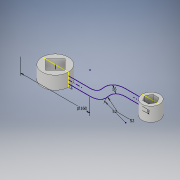
# Autodesk Inventor part: 練習三
Saved by Autodesk Inventor 2017 (Build 210142000, 142)
## iProperties
Part Number: 練習三
Material: 一般
Document SubType Name: Modeling
Designer: user
Density: 1 g/cm^3
Appearance: 預設
Author: user
Autodesk Inventor part; units mm, degrees
ref_plane "YZ Plane" through (0, 0, 0) normal (1, 0, 0) x (0, 1, 0)
ref_plane "XY Plane" through (0, 0, 0) normal (0, 0, 1) x (1, 0, 0)
sketch "草圖1" plane through (0, 0, 0) normal (0, 1, 0) x (-1, 0, 0)
  circle A0 centre (0, 0) radius 30
  line L0 (0, 22.6274) -> (-22.6274, 0)
  line L1 (-22.6274, 0) -> (0, -22.6274)
  line L2 (0, -22.6274) -> (22.6274, 0)
  line L3 (22.6274, 0) -> (0, 22.6274)
  line L4 (17.214, 3.8392) -> (-17.214, -3.8392) construction
  line L5 (-19.542, 13.3062) -> (19.542, -13.3062) construction
  line L6 (11.3137, -11.3137) -> (-26.3636, 26.3636)
  line L7 (-11.3137, -11.3137) -> (19.159, 19.159)
  dimension "d0" = 60
  dimension "d1" = 32
  dimension "d2" = 32
  constraints: 16 end point, 6 midpoint, 3 parallel, 3 point on line, 2 perpendicular, 1 centre point, 1 coincident, 1 other
  measures "d0" diameter of A0
  measures "d1" distance between parallel lines of L2 L0
  measures "d2" distance between parallel lines of L1 L3
extrude "擠出1" add sketch "草圖1" along normal blind 30
ref_plane "工作平面1" through (0, 71, 0) normal (0, 1, 0) x (1, 0, 0)
sketch "草圖2" plane through (0, 71, 0) normal (0, 1, 0) x (1, 0, 0)
  circle A0 centre (220, 0) radius 20
  line L0 (233.8564, 0) -> (226.9282, -12)
  line L1 (226.9282, -12) -> (213.0718, -12)
  line L2 (213.0718, -12) -> (206.1436, 0)
  line L3 (206.1436, 0) -> (213.0718, 12)
  line L4 (213.0718, 12) -> (226.9282, 12)
  line L5 (226.9282, 12) -> (233.8564, 0)
  point P0 (0, 0)
  dimension "d14" = 220
  dimension "d15" = 40
  dimension "d16" = 0
  dimension "d17" = 24
  constraints: 12 end point, 1 centre point, 1 coincident, 1 horizontal, 13 other
  measures "d14" distance of A0.centre point (0, 0)
  measures "d15" diameter of A0
  measures "d16" vertical distance of A0.centre point (0, 0)
  measures "d17" distance between parallel lines of L4 L1
extrude "擠出2" add sketch "草圖2" against normal blind 32
sketch "草圖3" plane through (0, 0, 0) normal (0, 0, 1) x (1, 0, 0)
  line L0 (-30, 0) -> (30, 0) projected
  line L1 (30, 7) -> (80, 7)
  line L2 (161.9756, 47) -> (200, 47)
  line L3 (200, 71) -> (200, 39) projected
  line L4 (200, 39) -> (240, 39) projected
  line L5 (30, 30) -> (-30, 30) projected
  line L6 (30, 0) -> (30, 30) projected
  line L7 (200, 71) -> (240, 71) projected
  arc A0 (161.9756, 47) -> (120.9878, 27) centre (161.9756, -5) ccw
  arc A1 (80, 7) -> (120.9878, 27) centre (80, 59) ccw
  line L8 (30, 15) -> (64.6593, 15)
  line L9 (200, 55) -> (179.5029, 55)
  line L10 (0, 30) -> (0, -21.4533)
  line L11 (30, 23) -> (80, 23)
  arc A2 (80, 23) -> (108.3762, 36.8462) centre (80, 59) ccw
  arc A3 (161.9756, 63) -> (108.3762, 36.8462) centre (161.9756, -5) ccw
  line L12 (161.9756, 63) -> (200, 63)
  dimension "d22" = 8
  dimension "d25" = 7
  dimension "d29" = 52
  dimension "d30" = 52
  dimension "d31" = 160
  dimension "d33" = 16
  constraints: 14 end point, 8 point on circle, 4 centre point, 3 midpoint, 3 tangent, 2 horizontal, 1 point on line, 1 vertical, 3 other
  measures "d22" distance between parallel lines of L2 L4
  measures "d25" distance between parallel lines of L1 L0
  measures "d29" radius of A1
  measures "d30" radius of A0
  measures "d31" diameter of L1.end L10
  measures "d33" radial gap between concentric circles of A0 A3
ref_plane "工作平面2" through (0, 35.75, 0) normal (0, 1, 0) x (-1, 0, 0)
